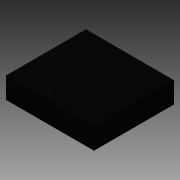
# Autodesk Inventor part: 2_2UH
Saved by Autodesk Inventor 2015 SP1 (Build 190203100, 203)
## iProperties
Created: 2015-10-19
Part Number: 2_2UH
Material: Generic
Document SubType Name: Modeling
Designer: Kartikye
Density: 1 g/cm^3
Appearance: IND_ELL3FU, 2_2UH
Author: Kartikye
Autodesk Inventor part; units mm, degrees
ref_plane "YZ Plane" through (0, 0, 0) normal (1, 0, 0) x (0, 1, 0)
ref_plane "XZ Plane" through (0, 0, 0) normal (0, 1, 0) x (-1, 0, 0)
ref_plane "XY Plane" through (0, 0, 0) normal (0, 0, 1) x (1, 0, 0)
sketch "IND_ELL3FU, 2_2UH_44" plane through (0, 0, 0) normal (0, 0, 1) x (1, 0, 0)
  line L0 (-2.0828, 1.8542) -> (2.0828, 1.8542)
  line L1 (2.0828, 1.8542) -> (2.0828, -1.9304)
  line L2 (2.0828, -1.9304) -> (-2.0828, -1.9304)
  line L3 (-2.0828, -1.9304) -> (-2.0828, 1.8542)
  constraints: 8 end point
extrude "Extrusion1" add sketch "IND_ELL3FU, 2_2UH_44" along normal blind 1
body "Solid1"
